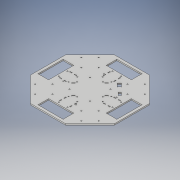
# Autodesk Inventor part: Base final final for sure this time
Saved by Autodesk Inventor 2019 (Build 230136000, 136)
## iProperties
Created: 2019-03-08
Part Number: Base final final for sure this time
Material: Generic
Document SubType Name: Modeling
Designer: jonas
Density: 1 g/cm^3
Appearance: Default
Author: jonas
Autodesk Inventor part; units mm, degrees
ref_plane "YZ Plane" through (0, 0, 0) normal (1, 0, 0) x (0, 1, 0)
ref_plane "XZ Plane" through (0, 0, 0) normal (0, 1, 0) x (-1, 0, 0)
ref_plane "XY Plane" through (0, 0, 0) normal (0, 0, 1) x (1, 0, 0)
sketch "Sketch2" plane through (0, 0, 0) normal (0, 1, 0) x (-1, 0, 0)
  line L0 (-54, -130.3675) -> (-130.3675, -54)
  line L1 (-130.3675, -54) -> (-130.3675, 54)
  line L2 (-130.3675, 54) -> (-54, 130.3675)
  line L3 (-54, 130.3675) -> (54, 130.3675)
  line L4 (54, 130.3675) -> (130.3675, 54)
  line L5 (130.3675, 54) -> (130.3675, -54)
  line L6 (130.3675, -54) -> (54, -130.3675)
  line L7 (54, -130.3675) -> (-54, -130.3675)
  line L8 (-39, -122.3675) -> (39, -122.3675)
  line L9 (39, -122.3675) -> (39, -89.3675)
  line L10 (39, -89.3675) -> (-39, -89.3675)
  line L11 (-39, -89.3675) -> (-39, -122.3675)
  line L12 (89.3675, -39) -> (122.3675, -39)
  line L13 (89.3675, 39) -> (89.3675, -39)
  line L14 (122.3675, -39) -> (122.3675, 39)
  line L15 (122.3675, 39) -> (89.3675, 39)
  line L16 (39, 89.3675) -> (39, 122.3675)
  line L17 (-39, 89.3675) -> (39, 89.3675)
  line L18 (39, 122.3675) -> (-39, 122.3675)
  line L19 (-39, 122.3675) -> (-39, 89.3675)
  line L20 (-89.3675, 39) -> (-122.3675, 39)
  line L21 (-89.3675, -39) -> (-89.3675, 39)
  line L22 (-122.3675, 39) -> (-122.3675, -39)
  line L23 (-122.3675, -39) -> (-89.3675, -39)
  circle A0 centre (-13.5, -83.3675) radius 1.6
  circle A1 centre (-13.5, -52.8675) radius 1.6
  circle A2 centre (13.5, -83.3675) radius 1.6
  circle A3 centre (13.5, -52.8675) radius 1.6
  circle A4 centre (83.3675, -13.5) radius 1.6
  circle A5 centre (83.3675, 13.5) radius 1.6
  circle A6 centre (52.8675, -13.5) radius 1.6
  circle A7 centre (52.8675, 13.5) radius 1.6
  circle A8 centre (13.5, 83.3675) radius 1.6
  circle A9 centre (-13.5, 83.3675) radius 1.6
  circle A10 centre (13.5, 52.8675) radius 1.6
  circle A11 centre (-13.5, 52.8675) radius 1.6
  circle A12 centre (-83.3675, 13.5) radius 1.6
  circle A13 centre (-83.3675, -13.5) radius 1.6
  circle A14 centre (-52.8675, 13.5) radius 1.6
  circle A15 centre (-52.8675, -13.5) radius 1.6
  line L24 (-10.3489, -46.5527) -> (-11.7631, -45.1385)
  line L25 (-11.7631, -45.1385) -> (-6.1062, -39.4817)
  line L26 (-6.1062, -39.4817) -> (-4.692, -40.8959)
  line L27 (-4.692, -40.8959) -> (-10.3489, -46.5527)
  circle A16 centre (44.7015, -71.6423) radius 1.6
  line L28 (-24.3422, -24.3422) -> (24.3422, 24.3422)
  line L29 (-24.3422, -24.3422) -> (44.5078, -24.3422) construction
  line L30 (16.6877, -16.6877) -> (-16.6877, 16.6877)
  line L31 (-46.5527, -10.3489) -> (-45.1385, -11.7631)
  line L32 (-45.1385, -11.7631) -> (-39.4817, -6.1062)
  line L33 (-39.4817, -6.1062) -> (-40.8959, -4.692)
  line L34 (-40.8959, -4.692) -> (-46.5527, -10.3489)
  line L35 (46.5527, 10.3489) -> (45.1385, 11.7631)
  line L36 (45.1385, 11.7631) -> (39.4817, 6.1062)
  line L37 (39.4817, 6.1062) -> (40.8959, 4.692)
  line L38 (40.8959, 4.692) -> (46.5527, 10.3489)
  line L39 (6.1062, 39.4817) -> (4.692, 40.8959)
  line L40 (10.3489, 46.5527) -> (11.7631, 45.1385)
  line L41 (11.7631, 45.1385) -> (6.1062, 39.4817)
  line L42 (4.692, 40.8959) -> (10.3489, 46.5527)
  line L43 (-32.0673, -65.4427) -> (-42.6739, -54.8361)
  line L44 (-42.6739, -54.8361) -> (-36.3099, -48.4722)
  line L45 (-36.3099, -48.4722) -> (-25.7033, -59.0788)
  line L46 (-25.7033, -59.0788) -> (-32.0673, -65.4427)
  line L47 (-56.9575, -40.5526) -> (-65.4427, -32.0673)
  line L48 (-65.4427, -32.0673) -> (-60.1394, -26.764)
  line L49 (-60.1394, -26.764) -> (-51.6542, -35.2493)
  line L50 (-51.6542, -35.2493) -> (-56.9575, -40.5526)
  line L51 (20.1657, -61.8405) -> (20.1657, -64.5905) construction
  line L52 (19.4157, -62.5905) -> (19.4157, -63.8405)
  line L53 (20.9157, -63.8405) -> (20.9157, -62.5905)
  arc A17 (20.9157, -62.5905) -> (19.4157, -62.5905) centre (20.1657, -62.5905) ccw
  arc A18 (19.4157, -63.8405) -> (20.9157, -63.8405) centre (20.1657, -63.8405) ccw
  arc A19 (62.5905, 20.9157) -> (62.5905, 19.4157) centre (62.5905, 20.1657) ccw
  line L54 (63.8405, 20.9157) -> (62.5905, 20.9157)
  line L55 (62.5905, 19.4157) -> (63.8405, 19.4157)
  arc A20 (63.8405, 19.4157) -> (63.8405, 20.9157) centre (63.8405, 20.1657) ccw
  line L56 (61.8405, 20.1657) -> (64.5905, 20.1657) construction
  arc A21 (-20.9157, 62.5905) -> (-19.4157, 62.5905) centre (-20.1657, 62.5905) ccw
  line L57 (-20.9157, 63.8405) -> (-20.9157, 62.5905)
  line L58 (-19.4157, 62.5905) -> (-19.4157, 63.8405)
  arc A22 (-19.4157, 63.8405) -> (-20.9157, 63.8405) centre (-20.1657, 63.8405) ccw
  line L59 (-20.1657, 61.8405) -> (-20.1657, 64.5905) construction
  arc A23 (-62.5905, -20.9157) -> (-62.5905, -19.4157) centre (-62.5905, -20.1657) ccw
  line L60 (-63.8405, -20.9157) -> (-62.5905, -20.9157)
  line L61 (-62.5905, -19.4157) -> (-63.8405, -19.4157)
  arc A24 (-63.8405, -19.4157) -> (-63.8405, -20.9157) centre (-63.8405, -20.1657) ccw
  line L62 (-61.8405, -20.1657) -> (-64.5905, -20.1657) construction
  circle A25 centre (31.75, -31.75) radius 1.6
  circle A26 centre (71.6423, -98.5831) radius 1.6
  circle A27 centre (71.6423, -44.7015) radius 1.6
  line L63 (78.3675, -17) -> (72.3675, -17)
  line L64 (72.3675, -17) -> (72.3675, -15)
  line L65 (72.3675, -15) -> (78.3675, -15)
  line L66 (78.3675, -15) -> (78.3675, -17)
  line L67 (63.8675, -17) -> (57.8675, -17)
  line L68 (57.8675, -17) -> (57.8675, -15)
  line L69 (57.8675, -15) -> (63.8675, -15)
  line L70 (63.8675, -15) -> (63.8675, -17)
  line L71 (86.8675, 0) -> (56.5675, 0)
  line L72 (78.3675, 17) -> (72.3675, 17)
  line L73 (72.3675, 17) -> (72.3675, 15)
  line L74 (72.3675, 15) -> (78.3675, 15)
  line L75 (78.3675, 15) -> (78.3675, 17)
  line L76 (63.8675, 17) -> (57.8675, 17)
  line L77 (57.8675, 17) -> (57.8675, 15)
  line L78 (57.8675, 15) -> (63.8675, 15)
  line L79 (63.8675, 15) -> (63.8675, 17)
  line L80 (-15, 63.8675) -> (-17, 63.8675)
  line L81 (-17, 63.8675) -> (-17, 57.8675)
  line L82 (-15, 57.8675) -> (-15, 63.8675)
  line L83 (-17, 57.8675) -> (-15, 57.8675)
  line L84 (17, 57.8675) -> (15, 57.8675)
  line L85 (0, 86.8675) -> (0, 56.5675)
  line L86 (15, 57.8675) -> (15, 63.8675)
  line L87 (17, 63.8675) -> (17, 57.8675)
  line L88 (15, 63.8675) -> (17, 63.8675)
  line L89 (17, 72.3675) -> (15, 72.3675)
  line L90 (15, 72.3675) -> (15, 78.3675)
  line L91 (15, 78.3675) -> (17, 78.3675)
  line L92 (17, 78.3675) -> (17, 72.3675)
  line L93 (-17, 72.3675) -> (-15, 72.3675)
  line L94 (-17, 78.3675) -> (-17, 72.3675)
  line L95 (-15, 72.3675) -> (-15, 78.3675)
  line L96 (-15, 78.3675) -> (-17, 78.3675)
  line L97 (-63.8675, -15) -> (-63.8675, -17)
  line L98 (-63.8675, -17) -> (-57.8675, -17)
  line L99 (-57.8675, -15) -> (-63.8675, -15)
  line L100 (-57.8675, -17) -> (-57.8675, -15)
  line L101 (-57.8675, 17) -> (-57.8675, 15)
  line L102 (-86.8675, 0) -> (-56.5675, 0)
  line L103 (-57.8675, 15) -> (-63.8675, 15)
  line L104 (-63.8675, 17) -> (-57.8675, 17)
  line L105 (-63.8675, 15) -> (-63.8675, 17)
  line L106 (-72.3675, 17) -> (-72.3675, 15)
  line L107 (-72.3675, 15) -> (-78.3675, 15)
  line L108 (-78.3675, 15) -> (-78.3675, 17)
  line L109 (-78.3675, 17) -> (-72.3675, 17)
  line L110 (-72.3675, -17) -> (-72.3675, -15)
  line L111 (-78.3675, -17) -> (-72.3675, -17)
  line L112 (-72.3675, -15) -> (-78.3675, -15)
  line L113 (-78.3675, -15) -> (-78.3675, -17)
  line L114 (15, -63.8675) -> (17, -63.8675)
  line L115 (17, -63.8675) -> (17, -57.8675)
  line L116 (15, -57.8675) -> (15, -63.8675)
  line L117 (17, -57.8675) -> (15, -57.8675)
  line L118 (-17, -57.8675) -> (-15, -57.8675)
  line L119 (0, -86.8675) -> (0, -56.5675)
  line L120 (-15, -57.8675) -> (-15, -63.8675)
  line L121 (-17, -63.8675) -> (-17, -57.8675)
  line L122 (-15, -63.8675) -> (-17, -63.8675)
  line L123 (-17, -72.3675) -> (-15, -72.3675)
  line L124 (-15, -72.3675) -> (-15, -78.3675)
  line L125 (-15, -78.3675) -> (-17, -78.3675)
  line L126 (-17, -78.3675) -> (-17, -72.3675)
  line L127 (17, -72.3675) -> (15, -72.3675)
  line L128 (17, -78.3675) -> (17, -72.3675)
  line L129 (15, -72.3675) -> (15, -78.3675)
  line L130 (15, -78.3675) -> (17, -78.3675)
  line L131 (78.7134, -105.6542) -> (111.5233, -138.4641)
  circle A28 centre (98.5831, -71.6423) radius 1.6
  circle A29 centre (98.5831, 71.6423) radius 1.6
  circle A30 centre (71.6423, 98.5831) radius 1.6
  circle A31 centre (44.7015, 71.6423) radius 1.6
  circle A32 centre (71.6423, 44.7015) radius 1.6
  circle A33 centre (-71.6423, 98.5831) radius 1.6
  circle A34 centre (-98.5831, 71.6423) radius 1.6
  circle A35 centre (-71.6423, 44.7015) radius 1.6
  circle A36 centre (-44.7015, 71.6423) radius 1.6
  circle A37 centre (-98.5831, -71.6423) radius 1.6
  circle A38 centre (-71.6423, -98.5831) radius 1.6
  circle A39 centre (-44.7015, -71.6423) radius 1.6
  circle A40 centre (-71.6423, -44.7015) radius 1.6
  circle A41 centre (0, -40) radius 1.6
  circle A42 centre (31.75, 31.75) radius 1.6
  circle A43 centre (40, 0) radius 1.6
  circle A44 centre (-31.75, 31.75) radius 1.6
  circle A45 centre (0, 40) radius 1.6
  circle A46 centre (-31.75, -31.75) radius 1.6
  circle A47 centre (-40, 0) radius 1.6
  point P0 (0, 0)
  point P1 (0, 0)
  point P2 (80704.7665, 0)
  point P3 (-80704.7665, 0)
  point P4 (0, 0)
  point P5 (0, 0)
  point P6 (0, 0)
  point P7 (0, 0)
  point P8 (0, 0)
  point P9 (0, 0)
  point P10 (20.1657, -63.2155)
  point P11 (63.2155, 20.1657)
  point P12 (-20.1657, 63.2155)
  point P13 (-63.2155, -20.1657)
  dimension "d5" = 8
  dimension "d6" = 33
  dimension "d7" = 15
  dimension "d8" = 15
  dimension "d11" = 360
  dimension "d13" = 78
  dimension "d16" = 6
  dimension "d18" = 30.5
  dimension "d21" = 360
  dimension "d24" = 2
  dimension "d25" = 8
  dimension "d29" = 3.2
  dimension "d41" = 3.2
  dimension "d48" = 68.85
  dimension "d49" = 45
  dimension "d50" = 47.2
  dimension "d51" = 23.6
  dimension "d52" = 9
  dimension "d53" = 15
  dimension "d56" = 68.95
  dimension "d57" = 23.6
  dimension "d58" = 68.95
  dimension "d59" = 23.6
  dimension "d60" = 7.5
  dimension "d61" = 12
  dimension "d62" = 2.75
  dimension "d63" = 1.5
  dimension "d66" = 360
  dimension "d83" = 3.2
  dimension "d90" = 3.2
  dimension "d106" = 5
  dimension "d107" = 1.5
  dimension "d108" = 2
  dimension "d109" = 6
  dimension "d110" = 5
  dimension "d111" = 1.5
  dimension "d112" = 6
  dimension "d113" = 2
  dimension "d116" = 360
  dimension "d128" = 10
  dimension "d129" = 48.1
  dimension "d131" = 38.1
  dimension "d134" = 360
  dimension "d138" = 3.2
  dimension "d141" = 360
  dimension "d145" = 27
  dimension "d146" = 63.5
  dimension "d148" = 40
  constraints: 272 end point, 48 centre point, 24 point on circle, 22 symmetric about line, 16 parallel, 12 point on line, 8 perpendicular, 6 midpoint, 5 horizontal, 4 coincident, 4 tangent, 1 collinear, 1 equal length, 1 equal radius, 340 other
  measures "d5" distance between parallel lines of L8 L7
  measures "d6" distance between parallel lines of L10 L8
  measures "d7" distance from line of L0.start L11
  measures "d8" distance from line of L6.end L9
  measures "d13" distance between parallel lines of L11 L9
  measures "d16" distance from line of A0.centre L10
  measures "d18" distance of A1.centre A0.centre
  measures "d24" distance between parallel lines of L25 L27
  measures "d25" distance between parallel lines of L26 L24
  measures "d29" diameter of A3
  measures "d41" diameter of A16
  measures "d48" distance of L28.start L28.end
  measures "d49" angle of L29 L28
  measures "d50" distance of L30.start L30.end
  measures "d51" distance between parallel lines of L28 L25
  measures "d52" distance between parallel lines of L45 L43
  measures "d53" distance between parallel lines of L44 L46
  measures "d56" distance between parallel lines of L30 L43
  measures "d57" distance between parallel lines of L28 L46
  measures "d58" distance between parallel lines of L47 L30
  measures "d59" distance between parallel lines of L48 L28
  measures "d60" distance between parallel lines of L47 L49
  measures "d61" distance between parallel lines of L48 L50
  measures "d62" distance of L51.start L51.end
  measures "d63" diameter of A18
  measures "d83" diameter of A25
  measures "d90" diameter of A26
  measures "d106" distance from line of L66 A4.centre
  measures "d107" distance from line of L65 A4.centre
  measures "d108" distance between parallel lines of L67 L69
  measures "d109" distance between parallel lines of L70 L68
  measures "d110" distance from line of A6.centre L68
  measures "d111" distance from line of A6.centre L69
  measures "d112" distance between parallel lines of L64 L66
  measures "d113" distance between parallel lines of L65 L63
  measures "d128" distance from line of A26.centre L6
  measures "d129" distance from line of L6 A16.centre
  measures "d131" distance from line of A28.centre L131
  measures "d138" diameter of A41
  measures "d145" distance of A0.centre A2.centre
  measures "d146" distance of A25.centre A42.centre
  measures "d148" distance of point (0, 0) A43.centre
extrude "Extrusion11" add sketch "Sketch2" along normal blind 4
equation "\"d8\" = d7"
body "Solid11"
